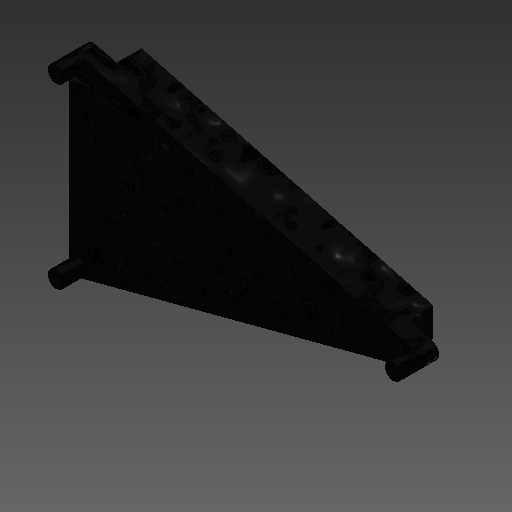
# Autodesk Inventor part: 3d_LM-Welding_Tooling - Top Adapter
Saved by Autodesk Inventor 2018.3 (Build 223284000, 284)
## iProperties
Created: 2026-01-23
Part Number: 3d_LM-Welding_Tooling - Top Adapter
Material: PA12 SLS 3D Print
Document SubType Name: Modeling
Designer: aca6
Density: 0.95 g/cm^3
Appearance: Black
Mass: 18.345 g
Surface Area: 66.8842 cm^2
Volume: 19.3105 cm^3
Manufacturer-1: {"Name": "MATERIALISE NV", "PartNumber": "3d_Welding_Tooling - Top Adapter", "Link": ""}
Manufacturer-2: {"Name": "BERNARDO HENAREJOS ORENES", "PartNumber": "3d_Welding_Tooling - Top Adapter", "Link": ""}
Manufacturer-3: {"Name": "", "PartNumber": "", "Link": ""}
Manufacturer-4: {"Name": "", "PartNumber": "", "Link": ""}
Manufacturer-5: {"Name": "", "PartNumber": "", "Link": ""}
Provider-1: {"Name": "", "PartNumber": "", "Link": ""}
Provider-2: {"Name": "", "PartNumber": "", "Link": ""}
Provider-3: {"Name": "", "PartNumber": "", "Link": ""}
Provider-4: {"Name": "", "PartNumber": "", "Link": ""}
Provider-5: {"Name": "", "PartNumber": "", "Link": ""}
Author: aca6
Comments: DIN-ISO-2768-mK
Autodesk Inventor part; units mm, degrees
ref_plane "YZ Plane" through (0, 0, 0) normal (1, 0, 0) x (0, 1, 0)
ref_plane "XZ Plane" through (0, 0, 0) normal (0, 1, 0) x (-1, 0, 0)
sketch "Sketch1" plane through (0, 0, 0) normal (0, 0, 1) x (1, 0, 0)
  circle A0 centre (-53.184, -21.25) radius 1.5 projected
  arc A1 (-60.184, 31.25) -> (-62.184, 29.25) centre (-60.184, 29.25) ccw projected
  line L0 (-62.184, -29.25) -> (-62.184, 29.25) projected
  arc A2 (-62.184, -29.25) -> (-60.184, -31.25) centre (-60.184, -29.25) ccw projected
  line L1 (-47.8192, -31.25) -> (-60.184, -31.25) projected
  line L2 (-47.8192, -31.25) -> (-47.8192, 31.25) projected
  line L3 (-47.8192, 31.25) -> (-60.184, 31.25) projected
  circle A3 centre (-53.184, 21.25) radius 1.5 projected
  circle A4 centre (27.484, 0) radius 1.5 projected
  circle A5 centre (-53.184, 21.25) radius 2
  circle A6 centre (-53.184, 21.25) radius 1 projected
  circle A7 centre (-53.184, -21.25) radius 1 projected
  circle A8 centre (-53.184, -21.25) radius 2
  circle A9 centre (27.484, 0) radius 2
  circle A10 centre (27.484, 0) radius 1 projected
  line L4 (-52.6745, 23.184) -> (27.9935, 1.934)
  line L5 (27.9935, -1.934) -> (-52.6745, -23.184)
  line L6 (-55.184, -21.25) -> (-55.184, 21.25)
  arc A11 (-52.6745, 23.184) -> (-55.184, 21.25) centre (-53.184, 21.25) ccw
  arc A12 (-55.184, -21.25) -> (-52.6745, -23.184) centre (-53.184, -21.25) ccw
  arc A13 (27.9935, -1.934) -> (27.9935, 1.934) centre (27.484, 0) ccw
  point P0 (0, 0)
  dimension "d0" = 4
  dimension "d1" = 4
  dimension "d2" = 4
  dimension "d3" = 2
  constraints: 6 centre point, 6 end point, 6 point on circle, 6 tangent, 3 coincident, 3 concentric, 2 equal radius, 1 vertical
  measures "d0" diameter of A5
  measures "d1" diameter of A8
  measures "d2" diameter of A9
  measures "d3" radius of A11
extrude "Extrusion1" add sketch "Sketch1" along normal blind 9 contours A0 | A5 | A9 | A8 | A3 | A4
extrude "Extrusion2" add sketch "Sketch1" along normal blind 4 contours L4 A9 L5 L2 | L2 L5 A8 L6 A5 L4
sketch "Sketch2" plane through (0, 0, 0) normal (0, 0, -1) x (-1, 0, 0)
  line L0 (-22.1808, 31.25) -> (-22.1808, -31.25) projected
  line L1 (47.8192, 31.25) -> (-22.1808, 31.25) projected
  line L2 (47.8192, -31.25) -> (47.8192, 31.25) projected
  line L3 (-22.1808, -31.25) -> (47.8192, -31.25) projected
  line L4 (47.8192, -21.905) -> (47.8192, 21.905)
  line L5 (47.8192, 21.905) -> (-22.1808, 3.4652)
  line L6 (-22.1808, 3.4652) -> (-22.1808, -3.4652)
  line L7 (-22.1808, -3.4652) -> (47.8192, -21.905)
  line L8 (52.6745, 23.184) -> (-27.9935, 1.934) projected
  line L9 (-27.9935, -1.934) -> (52.6745, -23.184) projected
  line L10 (47.7192, -21.8787) -> (47.7192, 21.8787)
  line L11 (47.7192, 21.7753) -> (-22.0808, 3.3882)
  line L12 (-22.0808, 3.4916) -> (-22.0808, -3.4916)
  line L13 (-22.0808, -3.3882) -> (47.7192, -21.7753)
  line L14 (47.7192, 21.7753) -> (47.7192, 21.8787)
  line L15 (-22.0808, 3.3882) -> (-22.0808, 3.4916)
  line L16 (47.8192, 21.905) -> (-22.1808, 3.4652)
  point P0 (0, 0)
  point P1 (-22.1808, 0)
  dimension "d8" = 0.1
  dimension "d11" = 0.1
  dimension "d12" = 0.1
  dimension "d13" = 0.1
  constraints: 22 end point, 13 point on line, 3 vertical, 2 collinear, 2 midpoint
  measures "d8" distance between parallel lines of L7 L13
  measures "d11" distance between parallel lines of L6 L12
  measures "d12" distance between parallel lines of L5 L11
  measures "d13" distance between parallel lines of L4 L10
ref_plane "Work Plane1" through (-47.8192, -31.25, -6) normal (0, 0, 1) x (1, 0, 0)
extrude "Extrusion3" add sketch "Sketch2" along normal up to surface (6 mm away) contours L5 L10 L11 L12 | L12 L13 L10 L7 | L11 L10 L13 L12
body "Solid1"
